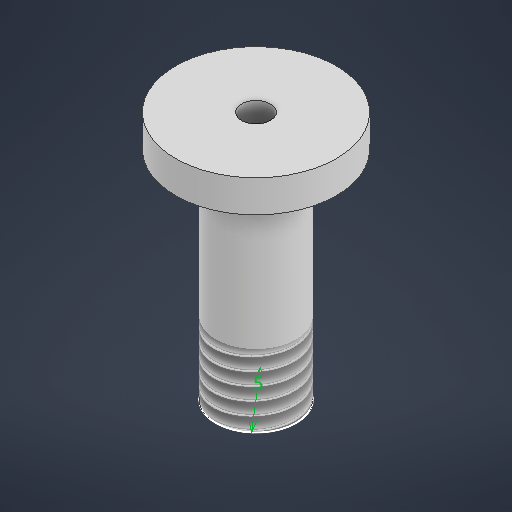
# Autodesk Inventor part: RadAdapterSchaft
Saved by Autodesk Inventor 2026.1 (Build 301233000, 233)
## iProperties
Created: 2025-10-13
Part Number: RadAdapterSchaft
Material: Generisch
Document SubType Name: Modeling
Designer: JurijLenz
Density: 1 g/cm^3
Appearance: Vorgabe
Author: JurijLenz
Autodesk Inventor part; units mm, degrees
ref_plane "YZ Plane" through (0, 0, 0) normal (1, 0, 0) x (0, 1, 0)
ref_plane "XZ Plane" through (0, 0, 0) normal (0, 1, 0) x (-1, 0, 0)
ref_plane "XY Plane" through (0, 0, 0) normal (0, 0, 1) x (1, 0, 0)
sketch "Skizze1" plane through (0, 0, 0) normal (0, 0, 1) x (1, 0, 0)
  circle A0 centre (0, 0) radius 2.5
  dimension "d1" = 5
  constraints: 2 coincident, 1 centre point
  measures "d1" diameter of A0
extrude "Extrusion1" add sketch "Skizze1" along normal blind 15.5
hole "Bohrung1" at (0, 0, 0) direction (0, 0, 1) diameter 1.8 end through all
thread "Gewinde1" size "M5x0.8" class "6g" standard "ANSI Metric M Profile" length 4.5
sketch "Skizze2" plane through (0, 0, 15.5) normal (0, 0, 1) x (1, 0, 0)
  circle A0 centre (0, 0) radius 0.9 projected
  circle A1 centre (0, 0) radius 5
  dimension "d13" = 10
  constraints: 1 centre point, 1 coincident
  measures "d13" diameter of A1
extrude "Extrusion2" add sketch "Skizze2" against normal blind 2
chamfer "Fasen1" distance 1 angle 45 1 edges at (-2.5, 0, 13.5)
